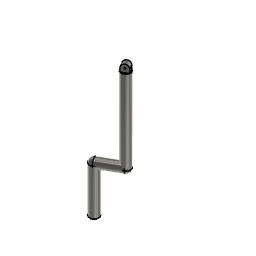
Tripod2 v1 (Autodesk Fusion 360 design; units mm, degrees)
Autodesk Fusion 360 part; units mm, degrees
sketch "Sketch1" plane through (-3, 5.1962, 0) normal (0.5, -0.866025, 0) x (0.866025, 0.5, 0)
  arc A0 (-70.01, 5) -> (-65.01, 0) centre (-65.01, 5) ccw
  line L0 (-65.01, 0) -> (-40.5586, 0)
  line L1 (-40.5586, 0) -> (-40.5586, 16)
  line L2 (-40.5586, 16) -> (-70.01, 16)
  line L3 (-70.01, 16) -> (-70.01, 5)
  circle A1 centre (-60.01, 8) radius 1.6
  arc A2 (-52.21, 8) -> (-67.81, 8) centre (-60.01, 8) ccw
  line L4 (-52.21, 8) -> (-52.21, -0.2)
  line L5 (-52.21, -0.2) -> (-67.81, -0.2)
  line L6 (-67.81, -0.2) -> (-67.81, 8)
  point P0 (-60.01, 8)
  dimension "d46" = 7.8
  dimension "d47" = 8.2
  dimension "d48" = 15.6
  constraint coincident P0 A1.centre
  constraint vertical L4
  constraint horizontal L5
  constraint vertical L6
  measures "d46" radius of A2
  measures "d47" distance of P0 L5
  measures "d48" distance of L4 L6
extrude "Extrude1" add sketch "Sketch1" along normal blind 11.8 contours A0 L0 A2 L4 L6 | A0 L0 L4 L5 L6 makes body 1
sketch "Sketch2" plane through (0, 0, -0.2) normal (0, 0, -1) x (1, 0, 0)
  line L0 (-61.7252, 28.7088) -> (-48.2152, 20.9088)
  line L1 (-48.2152, 20.9088) -> (-42.3152, 31.1279)
  line L2 (-42.3152, 31.1279) -> (-55.8252, 38.9279)
  line L3 (-55.8252, 38.9279) -> (-61.7252, 28.7088)
  circle A0 centre (-52.0202, 29.9184) radius 9.9
  circle A1 centre (-52.0202, 29.9184) radius 5.9
  point P0 (-52.0202, 29.9184)
  dimension "d51" = 5.9
  dimension "d52" = 7.8
  dimension "d53" = 19.8
  dimension "d54" = 11.8
  constraint coincident P0 A0.centre
  constraint concentric A0 A1
  measures "d51" distance of L2 P0
  measures "d52" distance of L3 P0
  measures "d53" diameter of A0
  measures "d54" diameter of A1
extrude "Extrude2" add sketch "Sketch2" along normal blind 180 separate body contours L0 L2 L3 A1 | L0 L1 L2 A1 | A0 makes body 2
sphere "SpherePrimitive1" add diameter 19.8 placed x (1, 0, 0) y (0, -1, 0) z (0, 0, -1) at (-52.0202, -29.9184, -180.2) separate body makes body 3
ref_plane "WorkPlane2" through (-43.4465, -24.9684, -90.2) normal (0.866025, 0.5, 0) x (0.5, -0.866025, 0)
sketch "Sketch6" plane through (0, 0, -180.2) normal (0, 0, -1) x (1, 0, 0)
  circle A0 centre (-52.0202, 29.9184) radius 5.9
  circle A1 centre (-52.0202, 29.9184) radius 9.9
  point P0 (-52.0202, 29.9184)
  constraint coincident P0 A0.centre
ref_plane "WorkPlane3" through (-51.9336, -29.8684, -90.2) normal (0.866025, 0.5, 0) x (0.5, -0.866025, 0)
cylinder "CylinderPrimitive1" add diameter 19.6 height -50 placed x (0.25, -0.433013, -0.866025) y (-0.433013, 0.75, -0.5) z (0.866025, 0.5, 0) at (-51.9336, -29.8684, -180.2) separate body makes body 4
sketch "Sketch8" plane through (-95.1849, -54.955, 0) normal (-0.866025, -0.5, 0) x (-0.5, 0.866025, 0)
  circle A0 centre (0.1, 180.2) radius 9.8
  circle A1 centre (0.1, 180.2) radius 5.9
  point P0 (0.1, 180.2)
  dimension "d66" = 11.8
  constraint concentric A0 A1
  constraint coincident P0 A0.centre
  measures "d66" diameter of A1
extrude "Extrude3" cut sketch "Sketch8" against normal blind 50 contours A1 bodies 2 3 4
sphere "SpherePrimitive3" add diameter 19.8 placed x (0.5, -0.866025, 0) y (0, 0, 1) z (-0.866025, -0.5, 0) at (-95.2349, -54.8684, -180.2) separate body makes body 5
ref_plane "WorkPlane6" through (-88.3827, -50.9123, -190) normal (0, 0, -1) x (-0.5, 0.866025, 0)
ref_plane "WorkPlane7" through (-88.3827, -50.9123, -180.2) normal (0, 0, -1) x (-0.5, 0.866025, 0)
sketch "Sketch19" plane through (-88.3827, -50.9123, -180.2) normal (0, 0, -1) x (1, 0, 0)
sketch "Sketch20" plane through (-88.3827, -50.9123, -180.2) normal (0, 0, -1) x (1, 0, 0)
  line L0 (31.5491, -29.5309) -> (41.3491, -12.5568)
  line L1 (-1.9522, 12.4432) -> (-11.7522, -4.5309)
cylinder "CylinderPrimitive3" add diameter 19.8 height 100 placed x (0, 1, 0) y (1, 0, 0) z (0, 0, -1) at (-95.2348, -54.8686, -180.2) separate body makes body 6
fillet "Fillet2" radius 2 1 edges at (-98.8148, -64.0986, -280.2) on bodies 6
sketch "Sketch22" plane through (0, 0, -280.2) normal (0, 0, -1) x (1, 0, 0)
  circle A0 centre (-95.2348, 54.8686) radius 7.9
  circle A1 centre (-95.2348, 54.8686) radius 5.9
  dimension "d86" = 11.8
  constraint concentric A0 A1
  measures "d86" diameter of A1
extrude "Extrude5" cut sketch "Sketch22" against normal blind 100 contours A1 bodies 4 5 6
